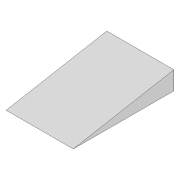
# Autodesk Inventor part: Finger_tip_wedge
Saved by Autodesk Inventor 2022 (Build 260153000, 153)
## iProperties
Created: 2022-08-29
Part Number: Finger_tip_wedge
Material: Generic
Document SubType Name: Modeling
Designer: dell
Density: 1 g/cm^3
Appearance: Default
Author: dell
Autodesk Inventor part; units mm, degrees
ref_plane "YZ Plane" through (0, 0, 0) normal (1, 0, 0) x (0, 1, 0)
ref_plane "XZ Plane" through (0, 0, 0) normal (0, 1, 0) x (-1, 0, 0)
ref_plane "XY Plane" through (0, 0, 0) normal (0, 0, 1) x (1, 0, 0)
sketch "Sketch2" plane through (0, 0, 0) normal (1, 0, 0) x (0, 1, 0)
  line L0 (0, 0) -> (5.4519, -30)
  line L1 (0, 0) -> (0, -30)
  line L2 (0, -30) -> (5.4519, -30)
  dimension "d0" = 10.3
  dimension "d1" = 30
  constraints: 6 end point, 1 perpendicular, 1 vertical
  measures "d0" angle of L1 L0
  measures "d1" distance from line of L0.start L2
extrude "Extrusion1" add sketch "Sketch2" along normal blind 20
body "Solid1"
